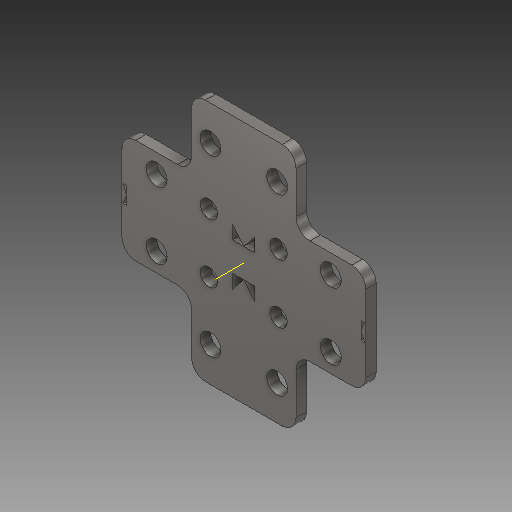
# Autodesk Inventor part: underbrink_base_lite
Saved by Autodesk Inventor 2019 (Build 230136000, 136)
## iProperties
Created: 2019-07-07
Part Number: underbrink_base_lite
Material: Stainless Steel
Document SubType Name: Modeling
Designer: Lino P
Density: 8 g/cm^3
Appearance: Semi-Polished
Mass: 70.8364 g
Surface Area: 75.4166 cm^2
Volume: 8.85455 cm^3
Author: Lino P
Autodesk Inventor part; units mm, degrees
ref_plane "YZ Plane" through (0, 0, 0) normal (1, 0, 0) x (0, 1, 0)
ref_plane "XZ Plane" through (0, 0, 0) normal (0, 1, 0) x (-1, 0, 0)
ref_plane "XY Plane" through (0, 0, 0) normal (0, 0, 1) x (1, 0, 0)
sketch "Sketch1" plane through (0, 0, 0) normal (0, 0, 1) x (1, 0, 0)
  line L0 (-336.1151, 0) -> (336.1151, 0) construction
  line L1 (15, 0) -> (50, 0) construction
  arc A0 (118.85, 219.94) -> (113.6034, 240) centre (-43.6266, 188.1614) ccw
  spline S0 degree 3 poles (118.85, 219.94) (128.5526, 163.9297) (111.383, 35.0272) (50, 0) knots 0 0 0 0 1 1 1 1
  line L2 (15, -15) -> (-15, -15)
  line L3 (-15, -15) -> (-15, 15)
  line L4 (-15, 15) -> (15, 15)
  line L5 (15, 15) -> (15, -15)
  line L6 (15, -15) -> (-15, 15) construction
  line L7 (-15, -15) -> (15, 15) construction
  line L8 (-32.5, -4.15) -> (32.5, -4.15) construction
  line L9 (32.5, -4.15) -> (32.5, 4.15) construction
  line L10 (32.5, 4.15) -> (-32.5, 4.15) construction
  line L11 (-32.5, 4.15) -> (-32.5, -4.15) construction
  line L12 (-32.5, -4.15) -> (32.5, 4.15) construction
  line L13 (32.5, -4.15) -> (-32.5, 4.15) construction
  arc A1 (15, 0) -> (50, 0) centre (32.5, 54.6766) ccw
  arc A2 (0, 15) -> (0, 50) centre (-54.6766, 32.5) ccw
  spline S1 degree 3 poles (-219.94, 118.85) (-163.9297, 128.5526) (-35.0272, 111.383) (0, 50) knots 0 0 0 0 1 1 1 1
  arc A3 (-219.94, 118.85) -> (-240, 113.6034) centre (-188.1614, -43.6266) ccw
  arc A4 (-15, 0) -> (-50, 0) centre (-32.5, -54.6766) ccw
  spline S2 degree 3 poles (-118.85, -219.94) (-128.5526, -163.9297) (-111.383, -35.0272) (-50, 0) knots 0 0 0 0 1 1 1 1
  arc A5 (-118.85, -219.94) -> (-113.6034, -240) centre (43.6266, -188.1614) ccw
  arc A6 (0, -15) -> (0, -50) centre (54.6766, -32.5) ccw
  spline S3 degree 3 poles (219.94, -118.85) (163.9297, -128.5526) (35.0272, -111.383) (0, -50) knots 0 0 0 0 1 1 1 1
  arc A7 (219.94, -118.85) -> (240, -113.6034) centre (188.1614, 43.6266) ccw
  point P0 (0, 0)
  point P1 (96.03, 57.2611)
  point P2 (119.66, 152.26)
  point P3 (119.6553, 152.2584)
  point P4 (0, 0)
  point P5 (-152.2584, 119.6553)
  point P6 (-57.2611, 96.03)
  point P7 (-15, 0)
  point P8 (-119.6553, -152.2584)
  point P9 (-96.03, -57.2611)
  point P10 (0, -15)
  point P11 (240, -113.6034)
  point P12 (152.2584, -119.6553)
  point P13 (57.2611, -96.03)
  point P14 (-15, 0)
  point P15 (-152.2584, 119.6553)
  point P16 (-57.2611, 96.03)
  point P17 (-119.6553, -152.2584)
  point P18 (-96.03, -57.2611)
  point P19 (152.2584, -119.6553)
  point P20 (57.2611, -96.03)
  dimension "d0" = 50
  dimension "d1" = 57.2611
  dimension "d2" = 96.03
  dimension "d3" = 119.66
  dimension "d6" = 118.85
  dimension "d12" = 240
  dimension "d38" = 65
  dimension "d39" = 8.3
  dimension "d61" = 360
  constraints: 26 end point, 16 point on circle, 8 centre point, 6 midpoint, 4 parallel, 3 coincident, 2 horizontal, 2 perpendicular, 2 point on line, 1 collinear, 61 other
  measures "d0" distance of point (0, 0) L1.end
  measures "d1" vertical distance of point (0, 0) point (96.03, 57.261)
  measures "d2" horizontal distance of point (0, 0) point (96.03, 57.261)
  measures "d3" horizontal distance of point (0, 0) point (119.66, 152.26)
  measures "d6" horizontal distance of point (0, 0) A0.start
  measures "d12" vertical distance of point (0, 0) A0.end
  measures "d38" distance of L10.end L9.end
  measures "d39" distance of L9.end L8.end
sketch "Sketch2" plane through (0, 0, 0) normal (1, 0, 0) x (0, 1, 0)
  point P0 (0, 0)
  point P1 (0, 0)
  point P2 (240, 0)
ref_plane "Work Plane1" through (15, 0, 0) normal (1, 0, 0) x (0, 1, 0)
sketch "Sketch3" plane through (15, 0, 0) normal (1, 0, 0) x (0, 1, 0)
  line L0 (-10, -0.5) -> (10, -0.5)
  line L1 (10, -0.5) -> (10, 0.5)
  line L2 (10, 0.5) -> (-10, 0.5)
  line L3 (-10, 0.5) -> (-10, -0.5)
  line L4 (-10, -0.5) -> (10, 0.5) construction
  line L5 (10, -0.5) -> (-10, 0.5) construction
  point P0 (0, 0)
  dimension "d8" = 20
  dimension "d9" = 1
  constraints: 12 end point, 2 midpoint, 2 parallel, 1 horizontal, 1 perpendicular
  measures "d8" distance of L2.end L1.end
  measures "d9" distance of L1.end L0.end
ref_plane "Work Plane2" through (52.6524, -10, -0.5) normal (0, 0, -1) x (-1, 0, 0)
sketch "Sketch4" plane through (52.6524, -10, -0.5) normal (0, 0, -1) x (-1, 0, 0)
  point P0 (52.6524, 10)
  point P1 (2.6524, 10)
  point P2 (-43.3776, 67.2611)
  point P3 (-67.0076, 162.26)
  point P4 (-66.1976, 229.94)
ref_plane "Work Plane3" through (15, -10, 0.5) normal (0, 0, 1) x (1, 0, 0)
sketch "Sketch5" plane through (15, -10, 0.5) normal (0, 0, 1) x (1, 0, 0)
  line L0 (17.5, 14.15) -> (-47.5, 14.15) construction
  line L1 (-47.5, 5.85) -> (17.5, 5.85) construction
  line L2 (-47.5, 14.15) -> (-47.5, 5.85) construction
  line L3 (17.5, 5.85) -> (17.5, 14.15) construction
  line L4 (0, -5) -> (20, -5)
  line L5 (20, -5) -> (20, 25)
  line L6 (20, 25) -> (0, 25)
  line L7 (0, 25) -> (0, -5)
  line L8 (0, 14.15) -> (20, 25) construction
  line L9 (20, 14.15) -> (0, 25) construction
  line L10 (0, -5) -> (20, 5.85) construction
  line L11 (20, -5) -> (0, 5.85) construction
  line L12 (10, 19.575) -> (10, 0.425) construction
  point P0 (-15, 10)
  point P1 (0, 25)
  point P2 (-30, 25)
  point P3 (-30, -5)
  dimension "d40" = 20
  dimension "d41" = 30
  constraints: 18 end point, 6 point on line, 3 parallel, 2 coincident, 2 midpoint, 1 horizontal, 1 perpendicular
  measures "d40" distance of L6.end L5.end
  measures "d41" distance of L5.end L4.end
ref_plane "Work Plane5" through (15, 15, 0.5) normal (0, 0, 1) x (1, 0, 0)
sketch "Sketch6" plane through (15, 15, 0.5) normal (0, 0, 1) x (1, 0, 0)
  circle A0 centre (81.03, 42.2611) radius 6.8 projected
  circle A1 centre (103.85, 204.94) radius 6.8 projected
  circle A2 centre (104.66, 137.26) radius 6.8 projected
  circle A3 centre (35, -15) radius 6.8 projected
  arc A4 (113.2428, 206.6719) -> (106.6941, 230.8772) centre (-58.6266, 173.1614) ccw projected
  line L0 (90.5128, 219.1228) -> (106.6941, 230.8772) projected
  arc A5 (94.5125, 203.2183) -> (90.5128, 219.1228) centre (-58.6266, 173.1614) ccw projected
  arc A6 (20, -8.1753) -> (29.677, -6.6675) centre (17.5, 39.6766) ccw projected
  line L1 (20, -8.1753) -> (20, 0) projected
  line L2 (20, 0) -> (0, 0) projected
  line L3 (0, 0) -> (0, -15) projected
  line L4 (-1.9583, -24.4011) -> (0, -15) projected
  arc A7 (-1.9583, -24.4011) -> (0, -24.9633) centre (17.5, 39.6766) ccw projected
  line L5 (0, -24.9633) -> (0, -30) projected
  line L6 (0, -30) -> (20, -30) projected
  line L7 (20, -30) -> (20, -27.2437) projected
  arc A8 (20, -27.2437) -> (37.8217, -24.1325) centre (17.5, 39.6766) ccw projected
  circle A9 centre (10, -24.575) radius 3 projected
  circle A10 centre (10, -5.425) radius 3 projected
  line L8 (0, -15) -> (0, 0) projected
  line L9 (0, 0) -> (-1.9583, 0)
  line L10 (-1.9583, 0) -> (-1.9583, -30)
  line L11 (-1.9583, -30) -> (0, -30)
  line L12 (0, -30) -> (0, 0)
  point P0 (-15, -15)
  constraints: 8 end point, 2 parallel, 1 horizontal, 1 perpendicular, 5 other
ref_plane "Work Plane4" through (15, 15, 0.5) normal (0, 0, 1) x (1, 0, 0)
sketch "Sketch7" plane through (15, 15, 0.5) normal (0, 0, 1) x (1, 0, 0)
  line L0 (-50, -30) -> (20, -30)
  line L1 (20, -30) -> (20, 0)
  line L2 (20, 0) -> (-50, 0)
  line L3 (-50, 0) -> (-50, -30)
  line L4 (-16, -30) -> (-14, -30)
  line L5 (-14, 0) -> (-16, 0)
  line L6 (20, -20) -> (20, -10)
  line L7 (-50, -10) -> (-50, -20)
  line L8 (20, 0) -> (20, -30)
  line L9 (20, -30) -> (0, -30)
  line L10 (-50, 0) -> (-30, 0)
  line L11 (-30, -30) -> (-50, -30)
  line L12 (-50, -30) -> (-50, 0)
  line L13 (20, -10) -> (20, 0)
  line L14 (20, 0) -> (0, 0)
  line L15 (0, -30) -> (20, -30) projected
  line L16 (20, -20) -> (20, -30)
  line L17 (20, -30) -> (0, -30)
  line L18 (-30, -30) -> (-16, -30)
  circle A0 centre (10, -5.425) radius 3 projected
  circle A1 centre (10, -24.575) radius 3 projected
  line L19 (-50, -15) -> (20, -15) construction
  circle A2 centre (-40, -5.425) radius 3
  circle A3 centre (-40, -24.575) radius 3
  line L20 (-48.7, -19.15) -> (18.7, -19.15) construction
  line L21 (-48.7, -10.85) -> (-48.7, -15) construction
  line L22 (-48.7, -19.15) -> (18.7, -10.85) construction
  line L23 (18.7, -19.15) -> (-48.7, -10.85) construction
  line L24 (-15, -10.85) -> (-18.212, -6.8756)
  line L25 (-15, -10.85) -> (-11.788, -6.8756)
  line L26 (-50, -19.15) -> (-50, -10.85)
  line L27 (20, -19.15) -> (18.7, -19.15)
  line L28 (20, -10.85) -> (20, -19.15)
  line L29 (18.7, -10.85) -> (-11.788, -10.85) construction
  line L30 (-18.212, -10.85) -> (-48.7, -10.85) construction
  line L31 (-18.212, -6.8756) -> (-11.788, -6.8756)
  line L32 (-48.7, -15) -> (-49.61, -12.5368)
  line L33 (-48.7, -15) -> (-49.61, -17.4632)
  line L34 (-49.61, -17.4632) -> (-49.61, -12.5368)
  line L35 (-18.212, -6.8756) -> (-11.788, -6.8756)
  line L36 (-11.788, -6.8756) -> (-11.788, -10.85)
  line L37 (-11.788, -10.85) -> (-18.212, -10.85)
  line L38 (-18.212, -10.85) -> (-18.212, -6.8756)
  line L39 (-15, -19.15) -> (-18.212, -23.1244)
  line L40 (-15, -19.15) -> (-11.788, -23.1244)
  line L41 (-18.212, -23.1244) -> (-11.788, -23.1244)
  line L42 (-18.212, -23.1244) -> (-11.788, -23.1244)
  line L43 (-11.788, -23.1244) -> (-11.788, -19.15)
  line L44 (-11.788, -19.15) -> (-18.212, -19.15)
  line L45 (-18.212, -19.15) -> (-18.212, -23.1244)
  line L46 (-15, 0) -> (-15, -30) construction
  line L47 (-49.61, -12.5368) -> (-48.7, -12.5368)
  line L48 (-48.7, -12.5368) -> (-48.7, -17.4632)
  line L49 (-48.7, -17.4632) -> (-49.61, -17.4632)
  line L50 (-49.61, -17.4632) -> (-49.61, -12.5368)
  line L51 (18.7, -15) -> (19.61, -12.5368)
  line L52 (18.7, -15) -> (19.61, -17.4632)
  line L53 (19.61, -17.4632) -> (19.61, -12.5368)
  line L54 (19.61, -12.5368) -> (18.7, -12.5368)
  line L55 (18.7, -12.5368) -> (18.7, -17.4632)
  line L56 (18.7, -17.4632) -> (19.61, -17.4632)
  line L57 (19.61, -17.4632) -> (19.61, -12.5368)
  circle A4 centre (-24.575, -40) radius 3
  circle A5 centre (-5.425, -40) radius 3
  circle A6 centre (10, -24.575) radius 3
  circle A7 centre (10, -5.425) radius 3
  circle A8 centre (-5.425, 10) radius 3
  circle A9 centre (-24.575, 10) radius 3
  line L58 (-30, 20) -> (0, 20)
  line L59 (0, 20) -> (0, 0)
  line L60 (0, 0) -> (-30, 0)
  line L61 (-30, 0) -> (-30, 20)
  line L62 (-30, 20) -> (0, 0) construction
  line L63 (0, 20) -> (-30, 0) construction
  line L64 (-30, -50) -> (0, -50)
  line L65 (0, -50) -> (0, -30)
  line L66 (-30, -30) -> (-30, -50)
  line L67 (-30, -50) -> (0, -50)
  line L68 (0, -50) -> (0, -30)
  line L69 (0, -30) -> (-30, -30)
  line L70 (-30, -30) -> (-30, -50)
  point P0 (-15, -15)
  point P1 (-15, 10)
  dimension "d63" = 2
  dimension "d72" = 6
  dimension "d73" = 6
  dimension "d77" = 67.4
  dimension "d78" = 8.3
  dimension "d84" = 70
  dimension "d91" = 360
  dimension "d93" = 30
  constraints: 140 end point, 17 symmetric about line, 15 parallel, 11 horizontal, 8 centre point, 8 midpoint, 8 point on line, 6 perpendicular, 4 coincident, 17 other
  measures "d63" distance of L5.end L5.start
  measures "d72" diameter of A2
  measures "d73" diameter of A3
  measures "d77" distance of L21.start L22.end
  measures "d78" distance of L22.end L20.end
  measures "d84" distance between parallel lines of L3 L1
  measures "d93" distance of L14.end L60.end
extrude "Extrusion7" add sketch "Sketch7" along normal blind 3 contours L3 L2 L1 L0 | L24 L31 L25 | L33 L34 L32 | L40 L41 L39 | L51 L53 L52
extrude "Extrusion8" add sketch "Sketch7" along normal blind 3 contours L61 L58 L59 L2
extrude "Extrusion9" add sketch "Sketch7" along normal blind 3 contours L0 L65 L64 L66
fillet "Fillet7" radius 4 12 edges at (15, 15, 2) (15, 35, 2) (35, 15, 2) (35, -15, 2) (15, -35, 2) (-15, -35, 2) (-15, -15, 2) (-35, -15, 2) (-35, 15, 2) (-15, 35, 2) (-15, 15, 2) (15, -15, 2)
sketch "Sketch8" plane through (15, 15, 3.5) normal (0, 0, 1) x (1, 0, 0)
  line L0 (-49.61, -12.5368) -> (-48.7, -12.5368) construction
  line L1 (19.61, -17.4632) -> (18.7, -17.4632) construction
  line L2 (-48.7, -12.5368) -> (18.7, -17.4632) construction
  line L3 (-48.7, -17.4632) -> (18.7, -12.5368) construction
  line L4 (-48.7, -12.5368) -> (18.7, -12.5368) construction
  line L5 (18.7, -12.5368) -> (18.7, -17.4632) construction
  line L6 (18.7, -17.4632) -> (-48.7, -17.4632) construction
  line L7 (-48.7, -17.4632) -> (-48.7, -12.5368) construction
  line L8 (-48.7, -12.5368) -> (-15, -12.5368) construction
  line L9 (-15, -12.5368) -> (-15, -17.4632) construction
  line L10 (-15, -17.4632) -> (-48.7, -17.4632) construction
  line L11 (-48.7, -17.4632) -> (-48.7, -12.5368) construction
  line L12 (-31.85, -17.4632) -> (-31.85, 4.3897) construction
  line L13 (-48.7, -15) -> (-15, -15) construction
  line L14 (-31.85, -6.5368) -> (-1.9543, -6.5368) construction
  line L15 (-48.7, -17.4632) -> (18.7, -17.4632)
  line L16 (18.7, -17.4632) -> (18.7, -12.5368)
  line L17 (18.7, -12.5368) -> (-48.7, -12.5368)
  line L18 (-48.7, -12.5368) -> (-48.7, -17.4632)
  point P0 (-25, -6.5368)
  point P1 (-25, -23.4632)
  point P2 (-5, -6.5368)
  point P3 (-5, -23.4632)
  dimension "d99" = 6
  dimension "d107" = 10
  constraints: 34 end point, 6 parallel, 5 horizontal, 4 midpoint, 3 perpendicular, 3 symmetric about line, 1 point on line, 1 vertical
  measures "d99" distance from line of L4 point (-25, -6.537)
  measures "d107" distance from line of L9 point (-25, -6.537)
hole "Hole4" at (-10, 8.4632, 3.5) at (-10, -8.4632, 3.5) at (10, -8.4632, 3.5) at (10, 8.4632, 3.5) direction (0, 0, -1) diameter 5 end through all
body "Solid2"
